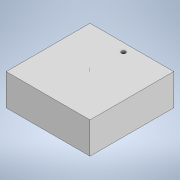
# Autodesk Inventor part: CajaBoya
Saved by Autodesk Inventor 2020 (Build 240168000, 168)
## iProperties
Created: 2021-10-16
Part Number: CajaBoya
Material: Genérico
Document SubType Name: Modeling
Designer: DANIEL
Density: 1 g/cm^3
Appearance: Valor por defecto
Author: DANIEL
Autodesk Inventor part; units mm, degrees
ref_plane "YZ Plane" through (0, 0, 0) normal (1, 0, 0) x (0, 1, 0)
ref_plane "XZ Plane" through (0, 0, 0) normal (0, 1, 0) x (-1, 0, 0)
ref_plane "XY Plane" through (0, 0, 0) normal (0, 0, 1) x (1, 0, 0)
sketch "Boceto1" plane through (0, 0, 0) normal (0, 1, 0) x (-1, 0, 0)
  line L0 (200, 200) -> (-200, 200)
  line L1 (-200, 200) -> (-200, -200)
  line L2 (-200, -200) -> (200, -200)
  line L3 (200, -200) -> (200, 200)
  point P0 (0, 0)
  dimension "d0" = 400
  dimension "L" = 400
  dimension "d2" = 200
  dimension "d3" = 200
  constraints: 8 end point, 2 parallel, 1 horizontal, 1 perpendicular
  measures "d0" distance between parallel lines of L1 L3
  measures "L" distance between parallel lines of L2 L0
  measures "d2" distance from line of L1 point (0, 0)
  measures "d3" distance from line of point (0, 0) L0
extrude "Extrusión1" add sketch "Boceto1" along normal blind 150
sketch "Boceto3" plane through (0, 150, 0) normal (0, 1, 0) x (1, 0, 0)
  circle A0 centre (0, 160) radius 10
  line L0 (200, 200) -> (-200, 200) projected
  point P0 (0, 0)
  dimension "d6" = 20
  dimension "d9" = 40
  constraints: 1 centre point
  measures "d6" diameter of A0
  measures "d9" distance from line of L0 A0.centre
extrude "Extrusión2" cut sketch "Boceto3" against normal blind 153.75
ref_plane "Plano de trabajo1" through (0, 0, 200) normal (1, 0, 0) x (0, 0, -1)
ref_plane "Plano de trabajo2" through (-200, 0, 0) normal (0, 0, 1) x (1, 0, 0)
equation "\"d0\" = L"
equation "\"d2\" = 0.5 * L"
equation "\"d3\" = 0.5 * L"
